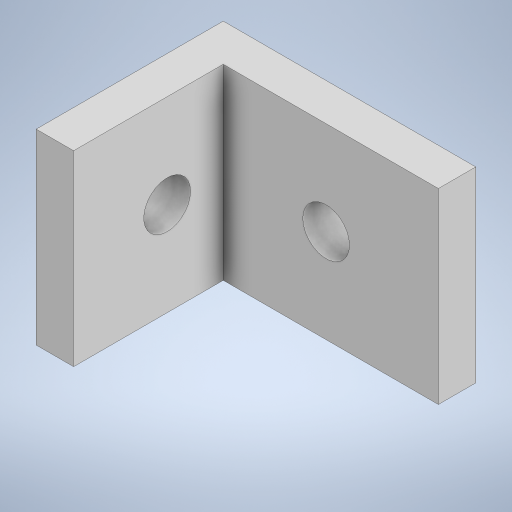
# Autodesk Inventor part: l-holder_2020
Saved by Autodesk Inventor 2024 (Build 280153000, 153)
## iProperties
Created: 2025-12-26
Part Number: l-holder_2020
Material: Generic
Document SubType Name: Modeling
Designer: schar
Density: 1 g/cm^3
Appearance: Default
Author: schar
Autodesk Inventor part; units mm, degrees
ref_plane "YZ Plane" through (0, 0, 0) normal (1, 0, 0) x (0, 1, 0)
ref_plane "XZ Plane" through (0, 0, 0) normal (0, 1, 0) x (-1, 0, 0)
ref_plane "XY Plane" through (0, 0, 0) normal (0, 0, 1) x (1, 0, 0)
sketch "Sketch1" plane through (0, 0, 0) normal (0, 1, 0) x (-1, 0, 0)
  line L0 (0, 0) -> (-20, 0)
  line L1 (-20, 0) -> (-20, 20)
  line L2 (-20, 20) -> (0, 20)
  line L3 (0, 20) -> (0, 0)
  line L4 (-20, 20) -> (-4, 20)
  line L5 (-4, 20) -> (-4, 4)
  line L6 (-4, 4) -> (-20, 4)
  line L7 (-20, 4) -> (-20, 20)
  dimension "d0" = 20
  dimension "d1" = 20
  dimension "d2" = 16
  dimension "d3" = 16
  constraints: 16 end point, 4 parallel, 2 horizontal, 2 perpendicular
  measures "d0" distance of L1.end L2.end
  measures "d1" distance of L0.end L1.end
  measures "d2" distance of L5.end L6.end
  measures "d3" distance of L4.end L5.end
extrude "Extrusion1" add sketch "Sketch1" along normal blind 20 contours L0 L1 L6 L5 L2 L3
sketch "Sketch2" plane through (0, 0, 0) normal (-1, 0, 0) x (0, 0, 1)
  line L0 (0, 0) -> (10, 0)
  line L1 (10, 0) -> (10, 10)
  line L2 (10, 10) -> (0, 10)
  line L3 (0, 10) -> (0, 0)
  circle A0 centre (10, 10) radius 2.5
  dimension "d6" = 10
  dimension "d7" = 10
  dimension "d8" = 5
  constraints: 8 end point, 2 parallel, 1 centre point, 1 coincident, 1 horizontal, 1 perpendicular
  measures "d6" distance of L2.end L1.end
  measures "d7" distance of L1.end L0.end
  measures "d8" diameter of A0
extrude "Extrusion2" cut sketch "Sketch2" against normal blind 20 contours A0 L2 L1 | L1 L2 A0
sketch "Sketch3" plane through (20, 0, 0) normal (0, 0, -1) x (-1, 0, 0)
  line L0 (16, 0) -> (0, 0) projected
  line L1 (0, 0) -> (5, 0)
  line L2 (5, 0) -> (5, 10)
  line L3 (5, 10) -> (0, 10)
  line L4 (0, 10) -> (0, 0)
  circle A0 centre (5, 10) radius 2.5
  point P0 (20, 0)
  dimension "d11" = 5
  dimension "d12" = 10
  dimension "d13" = 5
  constraints: 8 end point, 2 parallel, 1 centre point, 1 coincident, 1 horizontal, 1 perpendicular
  measures "d11" distance of L3.end L2.end
  measures "d12" distance of L2.end L1.end
  measures "d13" diameter of A0
extrude "Extrusion3" cut sketch "Sketch3" against normal blind 20 contours A0 L3 L2 | L2 L3 A0
sketch "Sketch4" plane through (20, 0, 4) normal (1, 0, 0) x (0, 0, -1)
  line L0 (4, 0) -> (-16, 0) projected
  line L1 (0, 0) -> (0, 20) projected
  line L2 (4, 0) -> (0, 0)
  line L3 (0, 0) -> (0, 20)
  line L4 (0, 20) -> (4, 20)
  line L5 (4, 20) -> (4, 0)
  constraints: 8 end point, 2 parallel, 1 horizontal, 1 perpendicular
extrude "Extrusion4" add sketch "Sketch4" along normal blind 7
body "Solid1"
